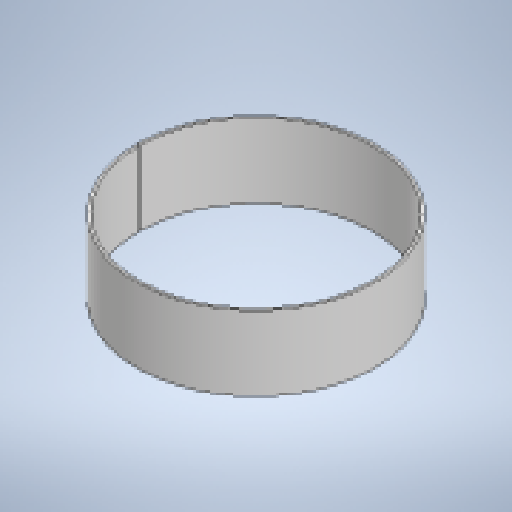
# Autodesk Inventor part: SLM 1603 accses hatch tube
Saved by Autodesk Inventor 2025.3 (Build 293356030, 356C)
## iProperties
Created: 2025-02-12
Part Number: SLM 1603 accses hatch tube
Material: Generic
Document SubType Name: Sheet Metal
Designer: pokla
Density: 1 g/cm^3
Flat Pattern Width: 169.687 cm
Flat Pattern Length: 17 cm
Flat Pattern Area: 2884.68 cm^2
Sheet Metal Rule: Default_mm
Sheet Metal Width: 1696,868 mm
Sheet Metal Length: 170,000 mm
Sheet Metal Area: 288467,593 mm^2
Appearance: Default
Mass: 1619.32 g
Surface Area: 5634.28 cm^2
Volume: 1619.32 cm^3
Author: pokla
Autodesk Inventor part; units mm, degrees
ref_plane "YZ Plane" through (0, 0, 0) normal (1, 0, 0) x (0, 1, 0)
ref_plane "XZ Plane" through (0, 0, 0) normal (0, 1, 0) x (-1, 0, 0)
ref_plane "XY Plane" through (0, 0, 0) normal (0, 0, 1) x (1, 0, 0)
sketch "Sketch1" plane through (0, 0, 0) normal (0, 1, 0) x (-1, 0, 0)
  line L0 (267.5, 120) -> (267.5, 0)
  line L1 (267.5, 0) -> (273.5, 0)
  line L2 (0, 0) -> (0, 109.131)
  line L3 (267.5, 120) -> (273.5, 120)
  line L4 (273.5, 0) -> (273.5, 120)
  line L5 (273.5, 0) -> (267.5, 0)
  line L6 (267.5, 0) -> (267.5, -50)
  line L7 (267.5, -50) -> (273.5, -50)
  line L8 (273.5, -50) -> (273.5, 0)
  point P0 (270.5, 0)
  point P1 (273.5, 0)
  point P2 (267.5, 0)
  dimension "d6" = 359.9
  dimension "d3" = 6
  dimension "d4" = 535
  dimension "d5" = 120
  dimension "d7" = 6
  dimension "d8" = 50
  constraints: 18 end point, 2 horizontal, 2 midpoint, 2 parallel, 2 perpendicular, 2 vertical, 1 horizontal alignment
  measures "d3" distance of L0.end L1.end
  measures "d4" diameter of L0 L2
  measures "d5" distance between parallel lines of L1 L3
  measures "d7" distance of L6.end L7.end
  measures "d8" distance of L7.end L5.start
revolve "Revolution1" add sketch "Sketch1" angle 359.9 about axis through (0, 0, 0) along (0, 0, 1)
sketch "Sketch2" plane through (0, 0, 0) normal (0, 1, 0) x (-1, 0, 0)
  circle A0 centre (0, -476) radius 476
  point P0 (0, 0)
  dimension "d6" = 359.9
  dimension "d9" = 952
  constraints: 2 vertical alignment, 2 other
extrude "Extrusion1" [suppressed]
equation "\"d4\" = Accsess_hatch_diameter"
equation "\"d5\" = Accsess_hatch_lenght"
equation "\"d7\" = d3"
equation "\"Accsess_hatch_lenght\" = 120"
equation "\"Accsess_hatch_diameter\" = 535"
equation "\"BendRadius\" = Thickness"
equation "\"BendReliefWidth\" = Thickness"
equation "\"BendReliefDepth\" = 0.5 * Thickness"
equation "\"CornerReliefSize\" = 4 * Thickness"
equation "\"MinimumRemnant\" = 2 * Thickness"
equation "\"TransitionRadius\" = BendRadius"
equation "\"JacobiRadiusSize\" = BendRadius"
equation "\"GapSize\" = Thickness"
equation "\"Thickness\" = 6"
body "Solid1"
